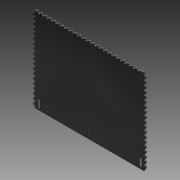
# Autodesk Inventor part: case_right
Saved by Autodesk Inventor 2014 (Build 180170000, 170)
## iProperties
Created: 2013-08-28
Part Number: case_right
Material: Polycarbonate, Clear
Document SubType Name: Modeling
Designer: Edward
Density: 1 g/cm^3
Appearance: Smoked - Light
Author: Edward
Autodesk Inventor part; units mm, degrees
ref_plane "YZ Plane" through (0, 0, 0) normal (1, 0, 0) x (0, 1, 0)
ref_plane "XZ Plane" through (0, 0, 0) normal (0, 1, 0) x (-1, 0, 0)
ref_plane "XY Plane" through (0, 0, 0) normal (0, 0, 1) x (1, 0, 0)
sketch "Sketch1" plane through (0, 0, 0) normal (0, 0, 1) x (1, 0, 0)
  line L0 (-253, -20) -> (-253, 20) projected
  line L1 (253, 20) -> (253, -20) projected
  line L2 (228, -26) -> (247, -26) projected
  line L3 (-107.5217, 353.1757) -> (-79.4293, 353.1757) projected
  line L4 (253, -26) -> (-253, -26)
  line L5 (-253, -26) -> (-253, 367.7)
  line L6 (-253, 367.7) -> (253, 367.7)
  line L7 (253, 367.7) -> (253, -26)
  point P0 (0, 0)
  dimension "d0" = 393.7
  constraints: 8 end point, 2 parallel, 1 horizontal, 1 perpendicular
  measures "d0" distance of L4.end L5.end
extrude "Extrusion1" add sketch "Sketch1" along normal blind 6.35
sketch "Sketch2" plane through (0, 0, 6.35) normal (0, 0, 1) x (1, 0, 0)
  line L0 (253, -26) -> (253, 367.7) projected
  line L1 (-253, 367.7) -> (-253, -26) projected
  circle A0 centre (-235, -12.5) radius 4.75 projected
  circle A1 centre (-235, 12.5) radius 4.75 projected
  circle A2 centre (235, -12.5) radius 4.75 projected
  circle A3 centre (235, 12.5) radius 4.75 projected
  line L2 (235, 12.5) -> (235, -12.5) construction
  line L3 (229, 12.5) -> (229, -12.5)
  line L4 (241, -12.5) -> (241, 12.5)
  arc A4 (241, 12.5) -> (229, 12.5) centre (235, 12.5) ccw
  arc A5 (229, -12.5) -> (241, -12.5) centre (235, -12.5) ccw
  line L5 (-235, -12.5) -> (-235, 12.5) construction
  line L6 (-229, -12.5) -> (-229, 12.5)
  line L7 (-241, 12.5) -> (-241, -12.5)
  arc A6 (-241, -12.5) -> (-229, -12.5) centre (-235, -12.5) ccw
  arc A7 (-229, 12.5) -> (-241, 12.5) centre (-235, 12.5) ccw
  point P0 (0, 0)
  point P1 (235, 0)
  point P2 (-235, 0)
  dimension "d3" = 12
  dimension "d4" = 12
  constraints: 16 end point, 8 point on circle, 8 tangent, 4 centre point, 4 parallel, 2 midpoint
  measures "d3" diameter of A5
  measures "d4" diameter of A7
extrude "Extrusion2" cut sketch "Sketch2" against normal blind 6.35 contours A0 | A1 | A2 | A3 | A4 L4 A5 L3 | A6 L7 A7 L6
sketch "Sketch3" plane through (0, 0, 6.35) normal (0, 0, 1) x (1, 0, 0)
  circle A0 centre (-195, -10) radius 2.75 projected
  circle A1 centre (-195, 10) radius 2.75 projected
  circle A2 centre (0, 10) radius 2.75 projected
  circle A3 centre (0, -10) radius 2.75 projected
  circle A4 centre (195, -10) radius 2.75 projected
  circle A5 centre (195, 10) radius 2.75 projected
  point P0 (0, 0)
extrude "Extrusion3" cut sketch "Sketch3" against normal blind 6.35
sketch "Sketch4" plane through (253, -26, 0) normal (1, 0, 0) x (0, 0, -1)
  line L0 (0, 393.7) -> (0, 0) projected
  line L1 (-6.35, 0) -> (-6.35, 393.7) projected
  line L2 (0, 11.85) -> (-6.35, 11.85)
  line L3 (-6.35, 11.85) -> (-6.35, 21.85)
  line L4 (-6.35, 21.85) -> (0, 21.85)
  line L5 (0, 21.85) -> (0, 11.85)
  line L6 (0, 0) -> (-6.35, 0) projected
  point P0 (0, 26)
  dimension "d9" = 10
  dimension "d15" = 11.85
  constraints: 8 end point, 2 parallel, 2 point on line, 1 horizontal, 1 perpendicular
  measures "d9" distance of L2.end L3.end
  measures "d15" distance between parallel lines of L6 L2
extrude "Extrusion4" add sketch "Sketch4" along normal blind 6.35 contours L0 L2 L1 L4
pattern_linear "Rectangular Pattern1" count 19 spacing 20 along (0, 1, 0) of "Extrusion4"
sketch "Sketch5" plane through (-253, -26, 0) normal (-1, 0, 0) x (0, 0, 1)
  line L0 (0, 0) -> (0, 393.7) projected
  line L1 (0, 0) -> (6.35, 0) projected
  line L2 (6.35, 393.7) -> (6.35, 0) projected
  line L3 (6.35, 11.85) -> (0, 11.85)
  line L4 (0, 11.85) -> (0, 21.85)
  line L5 (0, 21.85) -> (6.35, 21.85)
  line L6 (6.35, 21.85) -> (6.35, 11.85)
  point P0 (0, 26)
  dimension "d16" = 10
  dimension "d17" = 11.85
  constraints: 8 end point, 2 parallel, 2 point on line, 1 horizontal, 1 perpendicular
  measures "d16" distance of L3.end L4.end
  measures "d17" distance between parallel lines of L1 L3
extrude "Extrusion5" add sketch "Sketch5" along normal blind 6.35 contours L0 L5 L2 L3
pattern_linear "Rectangular Pattern2" count 19 spacing 20 along (0, 1, 0) of "Extrusion5"
sketch "Sketch6" plane through (0, 0, 6.35) normal (0, 0, 1) x (1, 0, 0)
  line L0 (253, 367.7) -> (-253, 367.7) projected
  line L1 (-238.6235, 367.7) -> (-228.6235, 367.7)
  line L2 (-228.6235, 367.7) -> (-228.6235, 361.35)
  line L3 (-228.6235, 361.35) -> (-238.6235, 361.35)
  line L4 (-238.6235, 361.35) -> (-238.6235, 367.7)
  point P0 (0, 0)
  dimension "d23" = 10
  dimension "d24" = 6.35
  constraints: 8 end point, 2 parallel, 1 horizontal, 1 perpendicular, 1 point on line
  measures "d23" distance of L2.end L3.end
  measures "d24" distance of L1.end L2.end
extrude "Extrusion6" cut sketch "Sketch6" against normal through all
pattern_linear "Rectangular Pattern3" count 24 spacing 20 along (1, 0, 0) of "Extrusion6"
body "Solid1"
